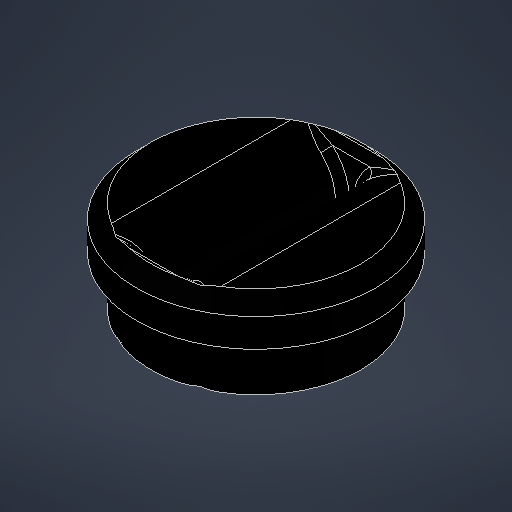
# Autodesk Inventor part: head_innter_top
Saved by Autodesk Inventor 2026.1 (Build 301233000, 233)
## iProperties
Created: 2026-04-17
Part Number: head_innter_top
Material: Aluminum 6061
Document SubType Name: Modeling
Designer: aaron
Density: 2.7 g/cm^3
Appearance: Aluminum - Flat
Author: aaron
Autodesk Inventor part; units mm, degrees
ref_plane "YZ Plane" through (0, 0, 0) normal (1, 0, 0) x (0, 1, 0)
ref_plane "XZ Plane" through (0, 0, 0) normal (0, 1, 0) x (-1, 0, 0)
ref_plane "XY Plane" through (0, 0, 0) normal (0, 0, 1) x (1, 0, 0)
sketch "Sketch1" plane through (0, 0, 0) normal (0, 0, 1) x (1, 0, 0)
  line L0 (0, 0) -> (0, 13)
  line L1 (0, 13) -> (14.9, 13)
  line L2 (14.9, 13) -> (16.9, 13)
  line L3 (16.9, 13) -> (16.9, 7)
  line L4 (16.9, 7) -> (14.9, 7)
  line L5 (14.9, 7) -> (14.9, 0)
  line L6 (14.9, 0) -> (0, 0)
  dimension "d0" = 13
  dimension "d3" = 14.9
  dimension "d4" = 2
  dimension "d5" = 6
  dimension "d6" = 2
  dimension "d7" = 7
  constraints: 14 end point, 3 perpendicular, 1 horizontal, 1 point on line, 1 vertical
  measures "d0" distance of L0.start L0.end
  measures "d3" distance of L0.end L1.end
  measures "d4" distance of L1.end L2.end
  measures "d5" distance of L2.end L3.end
  measures "d6" distance of L3.end L4.end
  measures "d7" distance of L4.end L5.end
revolve "Revolution1" add sketch "Sketch1" angle 360 about axis through (0, 0, 0) along (0, 1, 0)
sketch "Sketch2" plane through (0, 13, 0) normal (0, 1, 0) x (1, 0, 0)
  line L0 (1.25, 13.5) -> (-1.25, 13.5)
  line L1 (-1.25, 13.5) -> (-1.25, -13.5)
  line L2 (-1.25, -13.5) -> (1.25, -13.5)
  line L3 (1.25, -13.5) -> (1.25, 13.5)
  point P0 (0, 0)
  dimension "d9" = 2.5
  dimension "d10" = 27
  dimension "d11" = 13.5
  dimension "d12" = 1.25
  constraints: 8 end point, 2 parallel, 1 horizontal, 1 perpendicular
  measures "d9" distance between parallel lines of L3 L1
  measures "d10" distance of L2.end L0.start
  measures "d11" distance from line of point (0, 0) L2
  measures "d12" distance from line of L1 point (0, 0)
extrude "Extrusion1" cut sketch "Sketch2" against normal through all
fillet "Fillet1" radius 6.5 4 edges at (-1.25, 13, 0) (1.25, 13, 0) (-1.25, 0, 0) (1.25, 0, 0)
chamfer "Chamfer1" distance 2 angle 45 1 edges at (-16.9, 13, 0)
fillet "Fillet2" radius 1 4 edges at (0, 13, -13.5) (0, 13, 13.5) (0, 0, -13.5) (0, 0, 13.5)
sketch "Sketch4" plane through (0, 0, 0) normal (0, -1, 0) x (1, 0, 0)
  circle A0 centre (-11, -6) radius 1.25
  line L0 (0, 0) -> (0, -5.8419)
  line L1 (0, 0) -> (-3.1414, 0)
  circle A1 centre (-11, 6) radius 1.25
  circle A2 centre (11, -6) radius 1.25
  circle A3 centre (11, 6) radius 1.25
  dimension "d23" = 2.5
  dimension "d24" = 6
  dimension "d25" = 11
  dimension "d28" = 12
  dimension "d31" = 22
  constraints: 4 centre point, 4 end point, 2 horizontal, 2 vertical, 6 other
  measures "d23" diameter of A0
  measures "d24" distance from line of L1 A0.centre
  measures "d25" distance from line of A0.centre L0
  measures "d28" distance of A0.centre A1.centre
  measures "d31" distance of A0.centre A2.centre
extrude "Extrusion3" cut sketch "Sketch4" against normal blind 10
fillet "Fillet3" radius 1 12 edges at (-1.25, 6.5, 13.5) (-4.9902, 0.615, 13.5771) (-5.1556, 12.4598, 13.612) (5.1556, 12.4598, 13.612) (1.25, 6.5, 13.5) (4.9902, 0.615, 13.5771) (-5.1556, 12.4598, -13.612) (-1.25, 6.5, -13.5) (-4.9902, 0.615, -13.5771) (1.25, 6.5, -13.5) (4.9902, 0.615, -13.5771) (5.1556, 12.4598, -13.612)
equation "\"d0\" = d7 + d5"
equation "\"d11\" = 0.5 * d10"
equation "\"d12\" = 0.5 * d9"
body "Solid1"
